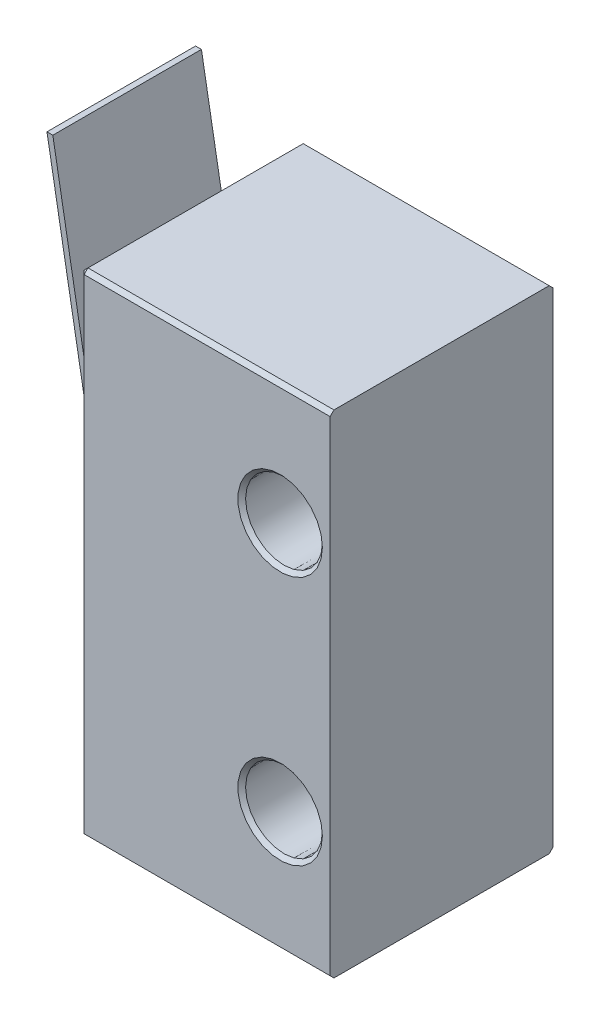
# Autodesk Inventor part: small-tact-switch
Saved by Autodesk Inventor 2016 (Build 200138000, 138)
## iProperties
Created: 2015-05-13
Part Number: small-tact-switch
Material: ABS Plastic
Document SubType Name: Modeling
Designer: as
Mass: 0.472885 g
Surface Area: 4.50599 cm^2
Volume: 0.446118 cm^3
Density: 1.06 g/cm^3
Appearance: Smooth - White
Author: as
Autodesk Inventor part; units mm, degrees
ref_plane "YZ Plane" through (0, 0, 0) normal (1, 0, 0) x (0, 1, 0)
ref_plane "XZ Plane" through (0, 0, 0) normal (0, 1, 0) x (-1, 0, 0)
ref_plane "XY Plane" through (0, 0, 0) normal (0, 0, 1) x (1, 0, 0)
sketch "Sketch2" plane through (0, 0, 0) normal (0, 0, 1) x (1, 0, 0)
  line L0 (0, 0) -> (-6.5, 0)
  line L1 (-6.5, 0) -> (-6.5, 12.8)
  line L2 (-6.5, 12.8) -> (0, 12.8)
  line L3 (0, 12.8) -> (0, 0)
  dimension "d0" = 6.5
  dimension "d1" = 12.8
  constraints: 8 end point, 2 parallel, 1 horizontal, 1 perpendicular
  measures "d0" distance of L1.end L2.end
  measures "d1" distance of L0.end L1.end
extrude "Extrusion1" add sketch "Sketch2" along normal blind 5.8
sketch "Sketch3" plane through (0, 0, 5.8) normal (0, 0, 1) x (1, 0, 0)
  line L0 (0, 6.4) -> (-6.5, 6.4)
  line L1 (0, 0) -> (0, 12.8) projected
  circle A0 centre (-1.3, 3.15) radius 1
  circle A1 centre (-1.3, 9.65) radius 1
  dimension "d4" = 6.5
  dimension "d5" = 6.5
  dimension "d6" = 1.3
  dimension "d7" = 2
  dimension "d8" = 12.8
  dimension "d9" = 0
  constraints: 2 centre point, 2 coincident, 2 end point, 2 symmetric about line, 1 horizontal, 1 other
  measures "d4" distance of L0.start L0.end
  measures "d5" diameter of point (-1.3, 3.15) L0
  measures "d6" distance from line of point (-1.3, 3.15) L1
  measures "d7" diameter of A0
  measures "d8" diameter of L1.end L0
  measures "d9" distance from line of L0.start L1
hole "Hole1" at (-1.3, 3.15, 5.8) at (-1.3, 9.65, 5.8) direction (0, 0, -1) diameter 2 end through all
sketch "Sketch4" plane through (-6.5, 0, 0) normal (-1, 0, 0) x (0, 0, 1)
  line L0 (0, 6.4) -> (6.5, 6.4)
  line L1 (0, 0) -> (5.8, 0) projected
  line L2 (2.9, 6.4) -> (2.9, 4.12) construction
  line L3 (2.9, 4.12) -> (0.2636, 4.12) construction
  line L4 (0.2636, 4.12) -> (5.5364, 4.12)
  line L5 (4.8, 4.32) -> (1, 4.32)
  line L6 (1, 4.32) -> (1, 3.92)
  line L7 (1, 3.92) -> (4.8, 3.92)
  line L8 (4.8, 3.92) -> (4.8, 4.32)
  line L9 (4.8, 4.32) -> (1, 3.92) construction
  line L10 (1, 4.32) -> (4.8, 3.92) construction
  dimension "d17" = 6.5
  dimension "d18" = 6.4
  dimension "d19" = 2.28
  dimension "d20" = 2.6364
  dimension "d21" = 5.2727
  dimension "d22" = 3.8
  dimension "d23" = 0.4
  constraints: 20 end point, 3 horizontal, 3 perpendicular, 2 midpoint, 2 parallel, 1 point on line
  measures "d17" distance of L0.start L0.end
  measures "d18" distance between parallel lines of L1 L0
  measures "d19" distance of L2.start L2.end
  measures "d20" distance of L2.end L3.end
  measures "d21" distance of L3.end L4.end
  measures "d22" distance of L7.end L6.end
  measures "d23" distance of L6.end L5.end
extrude "Extrusion2" add sketch "Sketch4" along normal blind 0.5
sketch "Sketch5" plane through (-6.5, 3.92, 4.8) normal (0, 0, 1) x (1, 0, 0)
  line L0 (-0.5, 0) -> (-0.5, 0.4) projected
  line L1 (0, 0) -> (-0.5, 0) projected
  arc A0 (-0.5, 0.4) -> (-0.5, 0) centre (-0.4899, 0.2) ccw
  point P0 (6.5, -3.92)
  constraints: 2 point on circle, 1 centre point
extrude "Extrusion3" add sketch "Sketch5" against normal up to surface (3.8 mm away)
chamfer "Chamfer1" distance 0.1 angle 45 10 edges at (-6.5, 0, 2.9) (-6.5, 6.4, 5.8) (-6.5, 6.4, 0) (-6.5, 12.8, 2.9) (-3.25, 12.8, 5.8) (-3.25, 0, 5.8) (-3.25, 0, 0) (-3.25, 12.8, 0) (-1.3, 4.15, 5.8) (-1.3, 10.65, 5.8)
sketch "Sketch6" plane through (0, 0, 0) normal (0, 0, -1) x (-1, 0, 0)
  line L0 (7.3899, 2.6671) -> (9.3, 13.5)
  line L1 (7.3899, 2.6671) -> (18.3899, 2.6671) construction
  line L2 (6.4, 12.7) -> (6.4, 0.1) projected
  line L3 (6.4, 1.9264) -> (4.4, 1.9264)
  line L4 (6.4, 1.9264) -> (8.4, 1.9264) construction
  arc A0 (6.4, 1.9264) -> (7.3899, 2.6671) centre (6.4, 2.9582) ccw
  line L5 (9.1477, 13.5) -> (7.2437, 2.7017)
  arc A1 (6.4, 2.0764) -> (7.2437, 2.7017) centre (6.4, 2.9582) ccw
  line L6 (6.4, 2.0764) -> (4.4, 2.0764)
  line L7 (4.4, 2.0764) -> (4.4, 1.9264)
  line L8 (9.3, 13.5) -> (9.1477, 13.5)
  line L9 (0, 0) -> (6.4, 0) projected
  dimension "d31" = 11
  dimension "d32" = 80
  dimension "d33" = 2
  dimension "d34" = 180
  dimension "d35" = 0.15
  dimension "d36" = 9.3
  dimension "d37" = 13.5
  dimension "d38" = 1.0318
  constraints: 16 end point, 4 point on circle, 2 centre point, 2 equal length, 2 horizontal, 2 perpendicular, 1 point on line, 1 tangent, 1 vertical, 2 other
  measures "d31" distance of L0.start L0.end
  measures "d32" angle of L1 L0
  measures "d33" distance of L3.start L3.end
  measures "d34" angle of L3 L4
  measures "d35" radial gap between concentric circles of A0 A1
  measures "d36" horizontal distance of L9.start L0.end
  measures "d37" distance from line of L9 L0.end
  measures "d38" radius of A0
extrude "Extrusion4" add sketch "Sketch6" against normal blind 3.8667
equation "\"d4\" = d0"
equation "\"d8\" = d1"
equation "\"d17\" = d0"
equation "\"d18\" = 0.5 * d1"
equation "\"d20\" = 0.454545 * d2"
equation "\"d21\" = 0.909091 * d2"
equation "\"d39\" = 0.666667 * d2"
equation "\"d2\" = 5.8"
body "Solid1"
